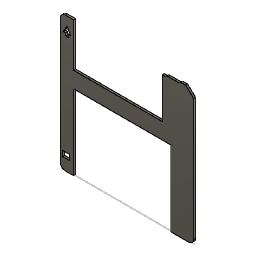
Floppy-Disk-Clock-Tutorial-Part2 (Autodesk Fusion 360 design; units mm, degrees)
Autodesk Fusion 360 part; units mm, degrees
note: some values were not read from the file. Set by a fixed rule: which sketch regions a step uses.
sketch "Sketch Floppy Disk" plane through (0, 0, 0) normal (0, 0, 1) x (1, 0, 0)
  line L0 (163.8, 0) -> (163.8, 155.9)
  line L1 (0, 165.8) -> (0, 0)
  line L2 (0, 165.8) -> (16.4, 165.8)
  line L3 (16.4, 165.8) -> (16.4, 112.1)
  line L4 (16.4, 112.1) -> (125.3, 112.1)
  line L5 (125.3, 112.1) -> (125.3, 161.8)
  line L6 (0, 0) -> (16.4, 0)
  line L7 (16.4, 0) -> (16.4, 92.4)
  line L8 (16.4, 92.4) -> (135.9, 92.4)
  line L9 (135.9, 92.4) -> (135.9, 0)
  line L10 (135.9, 0) -> (163.8, 0)
  line L11 (125.3, 161.8) -> (129.3, 161.8)
  line L12 (129.3, 161.8) -> (131.2, 163.45)
  line L13 (131.2, 163.45) -> (145.9, 163.45)
  line L14 (145.9, 163.45) -> (147.8, 165.1)
  line L15 (147.8, 165.1) -> (153.8, 165.1)
  line L16 (153.8, 165.1) -> (163.8, 155.9)
  line L17 (16.4, 164.3) -> (102.4, 164.3)
  line L18 (102.4, 164.3) -> (105, 161.8)
  line L19 (105, 161.8) -> (125.3, 161.8)
  line L20 (16.4, 1.5) -> (135.9, 1.5)
  line L21 (3, 20.2) -> (10.9, 20.2)
  line L22 (10.9, 20.2) -> (10.9, 13.6)
  line L23 (10.9, 13.6) -> (3, 13.6)
  line L24 (3, 13.6) -> (3, 20.2)
  line L25 (6.55, 143.8) -> (6.55, 147.1)
  line L26 (6.55, 147.1) -> (3.85, 147.1)
  line L27 (3.85, 147.1) -> (8.2, 155.1)
  line L28 (8.2, 155.1) -> (12.55, 147.1)
  line L29 (12.55, 147.1) -> (9.85, 147.1)
  line L30 (9.85, 147.1) -> (9.85, 143.8)
  line L31 (9.85, 143.8) -> (6.55, 143.8)
  line L32 (6.55, 143.8) -> (0, 143.8) construction
  line L33 (9.85, 143.8) -> (16.4, 143.8) construction
  circle A0 centre (157.8, 6) radius 6
  circle A1 centre (6, 6) radius 6
  circle A2 centre (6, 159.8) radius 6
  dimension "d7" = 16.4
  dimension "d8" = 27.9
  dimension "d9" = 119.5
  dimension "d10" = 108.9
  dimension "d12" = 53.7
  dimension "d13" = 92.4
  dimension "d14" = 14.7
  dimension "d15" = 6
  dimension "d16" = 4
  dimension "d17" = 10
  dimension "d18" = 9.2
  dimension "d19" = 1.5
  dimension "d20" = 165.1
  dimension "d21" = 86
  dimension "d22" = 24.3
  dimension "d23" = 49.7
  dimension "d24" = 1.5
  dimension "d25" = 6.6
  dimension "d26" = 7.9
  dimension "d27" = 13.6
  dimension "d28" = 3
  dimension "d29" = 3.3
  dimension "d30" = 3.3
  dimension "d31" = 2.7
  dimension "d32" = 8
  dimension "d33" = 22
  dimension "d34" = 165.8
  dimension "d37" = 6
  dimension "d38" = 6
  dimension "d39" = 6
  constraint vertical L0
  constraint vertical L1
  constraint coincident L1.end L6.start
  constraint perpendicular L1 L2
  constraint perpendicular L2 L3
  constraint perpendicular L1 L4
  constraint vertical L5
  constraint perpendicular L1 L6
  constraint perpendicular L6 L7
  constraint perpendicular L1 L8
  constraint perpendicular L8 L9
  constraint perpendicular L0 L10
  constraint equal L2 L6
  constraint collinear L6 L10
  constraint perpendicular L5 L11
  constraint perpendicular L5 L13
  constraint parallel L12 L14
  constraint parallel L13 L15
  constraint equal L12 L14
  constraint coincident L3 L17.start
  constraint perpendicular L3 L17
  constraint horizontal L19
  constraint coincident L7 L20.start
  constraint coincident L9 L20.end
  constraint perpendicular L9 L20
  constraint horizontal L21
  constraint vertical L22
  constraint horizontal L23
  constraint vertical L24
  constraint parallel L1 L25
  constraint perpendicular L1 L26
  constraint perpendicular L1 L29
  constraint perpendicular L26 L30
  constraint equal L25 L30
  constraint equal L26 L29
  constraint horizontal L31
  constraint equal L27 L28
  constraint coincident L1 L32.end
  constraint coincident L3 L33.end
  constraint equal L32 L33
  constraint horizontal L32
  constraint horizontal L33
  constraint tangent L10 A0
  constraint tangent L0 A0
  constraint tangent L1 A1
  constraint tangent L6 A1
  constraint tangent L2 A2
  constraint tangent L1 A2
  measures "d7" distance of L1.end L6.end
  measures "d8" distance of L0.start L9.end
  measures "d9" distance of L7.end L8.end
  measures "d10" distance of L3.end L4.end
  measures "d12" distance of L2.end L3.end
  measures "d13" distance of L6.end L7.end
  measures "d14" distance of L12.end L13.end
  measures "d15" distance of L14.end L15.end
  measures "d16" distance of L5.end L11.end
  measures "d17" horizontal distance of L0.end L15.end
  measures "d18" vertical distance of L0.end L15.end
  measures "d19" distance of L2.end L17.start
  measures "d20" vertical distance of L0.start L15.end
  measures "d21" distance of L17.start L17.end
  measures "d22" distance of L11.end L18.end
  measures "d23" distance of L4.end L5.end
  measures "d24" distance of L6.end L20.start
  measures "d25" distance of L21.start L23.end
  measures "d26" distance of L21.start L21.end
  measures "d27" distance of L6 L23
  measures "d28" distance of L1 L24
  measures "d29" horizontal distance of L25.start L30.end
  measures "d30" distance of L25.start L25.end
  measures "d31" distance of L25.end L26.end
  measures "d32" distance of L27.end L29
  measures "d33" distance of L2 L31
  measures "d34" distance of L1.end L1.start
  measures "d37" radius of A0
  measures "d38" radius of A1
  measures "d39" radius of A2
extrude "Extrude1" add sketch "Sketch Floppy Disk" along normal blind 2.5 contours L0 L1 L2 L3 L4 L5 L6 L7 L8 L9 L10 L11 L12 L13 L14 L15 L16 L25 L26 L27 L28 L29 L30 L31 A0 A1 A2 | A0 | A1 | L27 L28 A2 picked at (4.8212, 161.7351)
named bodies: "Body Front"
